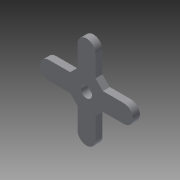
# Autodesk Inventor part: SimplifiedServoArm
Saved by Autodesk Inventor 2014 (Build 180170000, 170)
## iProperties
Created: 2013-09-08
Part Number: SimplifiedServoArm
Material: Generic
Document SubType Name: Modeling
Designer: Medrimonia
Density: 1 g/cm^3
Appearance: Default
ServoArmSpacing: 0.200 mm
ServoArmWidthRequired: 5.300 mm
ServoArmLengthRequired: 10.600 mm
ServoArmThickness: 1,900 mm
ServoArmHoleRequired: 3,000 mm
ServoArmInternFillet: 2,000 mm
ServoArmExternFillet: 2,450 mm
ServoArmHeadScrewTrace: 5,500 mm
ServoArmWidth: 4,900 mm
ServoArmLength: 10.200 mm
ServoArmHeadScrewThickness: 2,500 mm
Author: Medrimonia
Autodesk Inventor part; units mm, degrees
ref_plane "YZ Plane" through (0, 0, 0) normal (1, 0, 0) x (0, 1, 0)
ref_plane "XZ Plane" through (0, 0, 0) normal (0, 1, 0) x (-1, 0, 0)
ref_plane "XY Plane" through (0, 0, 0) normal (0, 0, 1) x (1, 0, 0)
sketch "Sketch2" plane through (0, 0, 0) normal (0, 1, 0) x (-1, 0, 0)
  line L0 (12.65, -2.45) -> (12.65, 2.45)
  line L1 (-12.65, 2.45) -> (-12.65, -2.45)
  line L2 (-12.65, -2.45) -> (12.65, 2.45) construction
  line L3 (12.65, -2.45) -> (-12.65, 2.45) construction
  line L4 (-2.45, -12.65) -> (2.45, -12.65)
  line L5 (2.45, 12.65) -> (-2.45, 12.65)
  line L6 (-2.45, -12.65) -> (2.45, 12.65) construction
  line L7 (2.45, -12.65) -> (-2.45, 12.65) construction
  line L8 (12.65, 2.45) -> (2.45, 2.45)
  line L9 (-2.45, 2.45) -> (-12.65, 2.45)
  line L10 (2.45, -12.65) -> (2.45, -2.45)
  line L11 (2.45, 2.45) -> (2.45, 12.65)
  line L12 (-12.65, -2.45) -> (-2.45, -2.45)
  line L13 (2.45, -2.45) -> (12.65, -2.45)
  line L14 (-2.45, 12.65) -> (-2.45, 2.45)
  line L15 (-2.45, -2.45) -> (-2.45, -12.65)
  circle A0 centre (0, 0) radius 1.5
  point P0 (0, 0)
  dimension "d7" = 4.9
  dimension "d8" = 4.9
  dimension "d9" = 10.2
  dimension "d10" = 3
  constraints: 32 end point, 10 parallel, 6 midpoint, 5 equal length, 4 perpendicular, 3 horizontal, 1 centre point
  measures "d7" distance of L5.start L5.end
  measures "d8" distance of L0.start L0.end
  measures "d9" distance of L0.end L8.end
  measures "d10" diameter of A0
extrude "Extrusion2" add sketch "Sketch2" along normal blind 1.9
fillet "Fillet1" radius 2.45 1 edges at (2.45, 0.95, 12.65)
fillet "Fillet2" radius 2.45 1 edges at (-2.45, 0.95, 12.65)
fillet "Fillet3" radius 2.45 1 edges at (12.65, 0.95, 2.45)
fillet "Fillet4" radius 2.45 1 edges at (12.65, 0.95, -2.45)
fillet "Fillet5" radius 2.45 1 edges at (2.45, 0.95, -12.65)
fillet "Fillet6" radius 2.45 1 edges at (-12.65, 0.95, 2.45)
fillet "Fillet7" radius 2.45 1 edges at (-12.65, 0.95, -2.45)
fillet "Fillet8" radius 2.45 1 edges at (-2.45, 0.95, -12.65)
chamfer "Chamfer1" distance 2 angle 45 1 edges at (-2.45, 0.95, -2.45)
chamfer "Chamfer2" distance 2 angle 45 1 edges at (2.45, 0.95, -2.45)
chamfer "Chamfer3" distance 2 angle 45 1 edges at (2.45, 0.95, 2.45)
chamfer "Chamfer4" distance 2 angle 45 1 edges at (-2.45, 0.95, 2.45)
equation "\"d7\" = ServoArmWidth"
equation "\"d8\" = ServoArmWidth"
equation "\"d9\" = ServoArmLength"
equation "\"d10\" = ServoArmHoleRequired"
equation "\"d11\" = ServoArmThickness"
equation "\"d13\" = ServoArmExternFillet"
equation "\"d14\" = ServoArmExternFillet"
equation "\"d15\" = ServoArmExternFillet"
equation "\"d16\" = ServoArmExternFillet"
equation "\"d17\" = ServoArmExternFillet"
equation "\"d18\" = ServoArmExternFillet"
equation "\"d19\" = ServoArmExternFillet"
equation "\"d20\" = ServoArmExternFillet"
equation "\"d21\" = ServoArmInternFillet"
equation "\"d24\" = ServoArmInternFillet"
equation "\"d27\" = ServoArmInternFillet"
equation "\"d30\" = ServoArmInternFillet"
equation "\"ServoArmWidth\" = 4.9"
equation "\"ServoArmSpacing\" = 0.2"
equation "\"ServoArmWidthRequired\" = ServoArmWidth + 2 * ServoArmSpacing"
equation "\"ServoArmLength\" = 10.2"
equation "\"ServoArmLengthRequired\" = ServoArmLength + 2 * ServoArmSpacing"
equation "\"ServoArmThickness\" = 1.9"
equation "\"ServoArmHoleRequired\" = 3"
equation "\"ServoArmInternFillet\" = 2"
equation "\"ServoArmExternFillet\" = 0.5 * ServoArmWidth"
equation "\"ServoArmHeadScrewTrace\" = 5.5"
equation "\"ServoArmHeadScrewThickness\" = 2.5"
body "Solid2"
